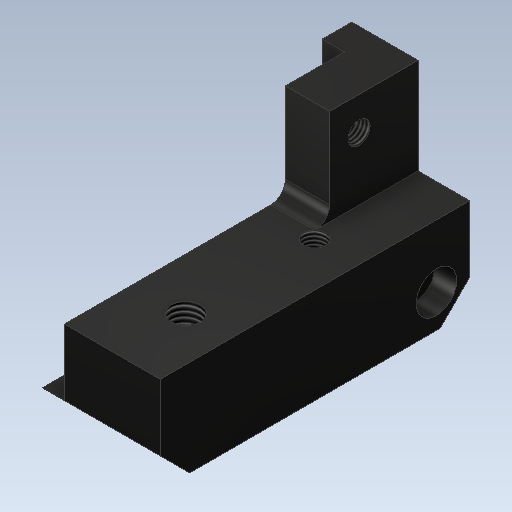
# Autodesk Inventor part: 34_ekstruder2
Saved by Autodesk Inventor 2020.2 (Build 242310000, 310)
## iProperties
Created: 2017-11-11
Part Number: 34_ekstruder2
Material: Ogólny
Document SubType Name: Modeling
Designer: Haras
Density: 1 g/cm^3
Appearance: Domyślna
Author: Haras
Autodesk Inventor part; units mm, degrees
ref_plane "YZ Plane" through (0, 0, 0) normal (1, 0, 0) x (0, 1, 0)
ref_plane "XZ Plane" through (0, 0, 0) normal (0, 1, 0) x (-1, 0, 0)
ref_plane "XY Plane" through (0, 0, 0) normal (0, 0, 1) x (1, 0, 0)
sketch "Szkic1" plane through (0, 0, 0) normal (1, 0, 0) x (0, 1, 0)
  line L0 (13, 21) -> (0, 21)
  line L1 (0, 21) -> (0, -21)
  line L2 (0, -21) -> (13, -21)
  line L3 (13, -21) -> (13, 21)
  line L4 (0, 0) -> (13, 0) construction
  dimension "d0" = 42
  dimension "d1" = 13
  constraints: 10 end point, 2 horizontal, 2 midpoint, 2 parallel, 1 perpendicular
  measures "d0" distance of L0.end L1.end
  measures "d1" distance of L1.end L2.end
extrude "Wyciągnięcie proste3" add sketch "Szkic1" along normal blind 16
chamfer "Faza1" distance 4 angle 45 2 edges at (8, 0, 21) (8, 0, -21)
sketch "Szkic6" plane through (0, 0, -17) normal (0, -1, 0) x (1, 0, 0)
  line L0 (0, -4) -> (16, -4) projected
  line L1 (0, 34) -> (0, 0) projected
  line L2 (16, 34) -> (16, 0) projected
  point P0 (0, 17)
  point P1 (10, 11)
  dimension "d28" = 15
  dimension "d53" = 6
  measures "d28" distance from line of L0 point (10, 11)
  measures "d53" distance from line of L2 point (10, 11)
hole "Otwór2" at (10, 0, -6) direction (0, 1, 0) diameter 3 end through all
sketch "Szkic7" plane through (0, 0, -17) normal (0, -1, 0) x (1, 0, 0)
  line L0 (16, 38) -> (0, 38) projected
  circle A0 centre (10, 11) radius 1.5 projected
  point P0 (0, 17)
  point P1 (10, 28.5)
  dimension "d37" = 9.5
  constraints: 1 vertical alignment
  measures "d37" distance from line of L0 point (10, 28.5)
hole "Otwór3" at (10, 0, 11.5) direction (0, 1, 0) diameter 4 end through all
thread "Gwint2" size "M4x0.7" class "6H" standard "ANSI Metric M Profile" full length
sketch "Szkic8" plane through (0, 0, 0) normal (-1, 0, 0) x (0, 0, 1)
  line L0 (21, 13) -> (-17, 13)
  line L1 (-17, 13) -> (-17, 9)
  line L2 (-12, 4) -> (21, 4)
  line L3 (21, 4) -> (21, 13)
  line L4 (17, 0) -> (-17, 0) projected
  line L5 (-21, 4) -> (-21, 13) projected
  line L6 (-12, 4) -> (-17, 9)
  point P0 (0, 0)
  point P1 (-17, 4)
  dimension "d55" = 4
  dimension "d56" = 4
  dimension "d59" = 5
  dimension "d60" = 5
  constraints: 10 end point, 2 parallel, 2 point on line, 1 horizontal, 1 perpendicular
  measures "d55" distance between parallel lines of L2 L4
  measures "d56" distance between parallel lines of L5 L1
  measures "d59" distance of L2.start point (-17, 4)
  measures "d60" distance of L1.end point (-17, 4)
extrude "Wyciągnięcie proste5" cut sketch "Szkic8" against normal blind 3
sketch "Szkic9" plane through (16, 0, 0) normal (1, 0, 0) x (0, 0, -1)
  line L0 (-17, 0) -> (17, 0) projected
  line L1 (21, 4) -> (21, 13) projected
  point P0 (0, 0)
  point P1 (16.5, 4.5)
  dimension "d63" = 4.5
  dimension "d64" = 4.5
  measures "d63" distance from line of L0 point (16.5, 4.5)
  measures "d64" distance from line of L1 point (16.5, 4.5)
hole "Otwór4" at (16, 4.5, -16.5) direction (-1, 0, 0) diameter 3 end through all
thread "Gwint5" size "M3x0.5" class "6H" standard "ANSI Metric M Profile" full length
sketch "Szkic10" plane through (16, 0, 0) normal (1, 0, 0) x (0, 0, -1)
  line L0 (21, 13) -> (-21, 13) projected
  line L1 (21, 13) -> (9, 13)
  line L2 (9, 13) -> (9, 26)
  line L3 (9, 26) -> (21, 26)
  line L4 (21, 26) -> (21, 13)
  point P0 (0, 0)
  dimension "d74" = 12
  dimension "d75" = 13
  constraints: 8 end point, 2 parallel, 1 horizontal, 1 perpendicular
  measures "d74" distance of L2.end L3.end
  measures "d75" distance of L3.end L0.start
extrude "Wyciągnięcie proste6" add sketch "Szkic10" against normal up to surface (16 mm away)
sketch "Szkic11" plane through (0, 0, 0) normal (-1, 0, 0) x (0, 0, 1)
  line L0 (-17, 9) -> (-17, 13) projected
  line L1 (-9, 26) -> (-21, 26) projected
  line L2 (-17, 13) -> (-9, 13)
  line L3 (-9, 13) -> (-9, 26)
  line L4 (-9, 26) -> (-17, 26)
  line L5 (-17, 26) -> (-17, 13)
  point P0 (0, 0)
  constraints: 8 end point, 2 parallel, 1 horizontal, 1 perpendicular
extrude "Wyciągnięcie proste7" cut sketch "Szkic11" against normal up to surface (3 mm away)
fillet "Zaokrąglenie2" radius 2 1 edges at (9.5, 13, -9)
sketch "Szkic12" plane through (16, 0, 0) normal (1, 0, 0) x (0, 0, -1)
  circle A0 centre (16.5, 4.5) radius 1.5 projected
  circle A1 centre (16.5, 4.5) radius 2.75
  point P0 (0, 0)
  dimension "d83" = 1.25
  constraints: 1 centre point
  measures "d83" radial gap between concentric circles of A0 A1
extrude "Wyciągnięcie proste8" cut sketch "Szkic12" against normal blind 3
sketch "Szkic13" plane through (16, 0, 0) normal (1, 0, 0) x (0, 0, -1)
  line L0 (7, 13) -> (-21, 13) projected
  line L1 (21, 4) -> (21, 26) projected
  line L2 (7, 13) -> (21, 13)
  line L3 (21, 13) -> (21, 26)
  line L4 (21, 26) -> (7, 26)
  line L5 (7, 26) -> (7, 13)
  point P0 (0, 0)
  constraints: 8 end point, 2 parallel, 1 horizontal, 1 perpendicular
extrude "Wyciągnięcie proste9" cut sketch "Szkic13" against normal blind 7
thread "Gwint7" size "M3x0.5" class "6H" standard "ANSI Metric M Profile" full length
sketch "Szkic14" plane through (9, 0, 0) normal (1, 0, 0) x (0, 0, -1)
  line L0 (21, 26) -> (21, 13) projected
  line L1 (9, 26) -> (21, 26) projected
  point P0 (0, 0)
  point P1 (13, 21.5)
  dimension "d90" = 8
  dimension "d91" = 4.5
  measures "d90" distance from line of L0 point (13, 21.5)
  measures "d91" distance from line of L1 point (13, 21.5)
hole "Otwór5" at (9, 21.5, -13) direction (-1, 0, 0) diameter 3 end through all
thread "Gwint8" size "M3x0.5" class "6H" standard "ANSI Metric M Profile" full length
equation "\"d60\" = d59"
